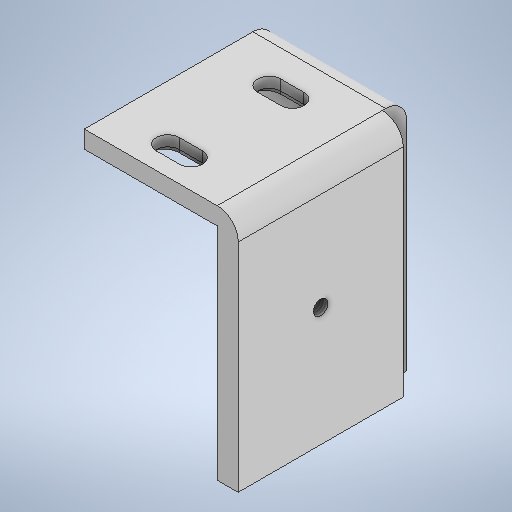
# Autodesk Inventor part: TS_Adapter_Greifer_int
Saved by Autodesk Inventor 2025.1 (Build 291241000, 241)
## iProperties
Created: 2025-06-16
Part Number: TS_Adapter_Greifer_int
Material: Generisch
Document SubType Name: Modeling
Designer: tino
Density: 1 g/cm^3
Appearance: Vorgabe
Author: tino
Autodesk Inventor part; units mm, degrees
ref_plane "YZ Plane" through (0, 0, 0) normal (1, 0, 0) x (0, 1, 0)
ref_plane "XZ Plane" through (0, 0, 0) normal (0, 1, 0) x (-1, 0, 0)
ref_plane "XY Plane" through (0, 0, 0) normal (0, 0, 1) x (1, 0, 0)
sketch "Skizze1" plane through (0, 0, 0) normal (0, 0, 1) x (1, 0, 0)
  line L0 (-19, 27.1) -> (19, 27.1)
  line L1 (19, 27.1) -> (19, -27.1)
  line L2 (19, -27.1) -> (-19, -27.1)
  line L3 (-19, -27.1) -> (-19, 27.1)
  line L4 (0, 37.94) -> (0, -37.94) projected
  line L5 (-26.6, 0) -> (26.6, 0) projected
  point P0 (0, 0)
  dimension "d0" = 38
  dimension "d1" = 54.2
  dimension "d46" = 19
  dimension "d47" = 27.1
  constraints: 8 end point, 2 parallel, 1 horizontal, 1 perpendicular
  measures "d0" distance of L1.end L2.end
  measures "d1" distance of L2.end L0.start
  measures "d46" distance between parallel lines of L3 L4
  measures "d47" distance between parallel lines of L5 L2
extrude "Extrusion1" add sketch "Skizze1" along normal blind 63
sketch "Skizze2" plane through (0, 0, 63) normal (0, 0, 1) x (1, 0, 0)
  line L0 (-19, -27.1) -> (19, -27.1) projected
  line L1 (-19, -27.1) -> (19, -27.1)
  line L2 (19, -27.1) -> (19, 21.1)
  line L3 (19, 21.1) -> (-19, 21.1)
  line L4 (-19, 21.1) -> (-19, -27.1)
  line L5 (-19, 27.1) -> (-19, -27.1) projected
  line L6 (19, 27.1) -> (-19, 27.1) projected
  point P0 (0, 0)
  dimension "d4" = 38
  dimension "d6" = 6
  constraints: 8 end point, 2 parallel, 1 collinear, 1 horizontal, 1 perpendicular, 1 point on line
  measures "d4" distance of L2.end L3.end
  measures "d6" distance between parallel lines of L6 L3
extrude "Extrusion2" cut sketch "Skizze2" against normal through all
sketch "Skizze6" plane through (-19, 27.1, 0) normal (0, 1, 0) x (1, 0, 0)
  line L0 (38, -63) -> (0, -63) projected
  line L1 (38, 0) -> (0, 0) projected
  line L2 (19, 12.6) -> (19, -75.6) projected
  point P0 (19, 0)
  point P1 (19, -44)
  point P2 (19, -19)
  dimension "d48" = 25
  dimension "d49" = 63
  dimension "d50" = 19
  constraints: 1 point on line, 1 vertical alignment
  measures "d48" distance of point (19, -19) point (19, -44)
  measures "d49" distance between parallel lines of L0 L1
  measures "d50" distance from line of L1 point (19, -19)
hole "Bohrung4" at (0, 27.1, 44) at (0, 27.1, 19) direction (0, -1, 0) diameter 5 depth 2.5
sketch "Skizze13" plane through (-19, 21.1, 63) normal (0, -1, 0) x (1, 0, 0)
  line L0 (38, 0) -> (38, -63) projected
  line L1 (0, -63) -> (0, 0) projected
  line L2 (38, -63) -> (0, -63) projected
  line L3 (0, 0) -> (38, 0) projected
  point P0 (19, -63)
  point P1 (7.6, -21.5)
  point P2 (27.6, -21.5)
  point P3 (27.6, -41.5)
  point P4 (7.6, -41.5)
  dimension "d102" = 20
  dimension "d103" = 20
  dimension "d104" = 38
  dimension "d105" = 7.6
  dimension "d106" = 63
  dimension "d107" = 21.5
  constraints: 2 horizontal alignment, 2 vertical alignment
  measures "d102" distance of point (27.6, -21.5) point (7.6, -21.5)
  measures "d103" distance of point (27.6, -21.5) point (27.6, -41.5)
  measures "d104" distance between parallel lines of L0 L1
  measures "d105" distance from line of L1 point (7.6, -41.5)
  measures "d106" distance between parallel lines of L2 L3
  measures "d107" distance from line of L2 point (27.6, -41.5)
hole "Bohrung6" at (-11.4, 21.1, 41.5) at (8.6, 21.1, 41.5) at (8.6, 21.1, 21.5) at (-11.4, 21.1, 21.5) direction (0, 1, 0) diameter 4.5 end through all counterbore diameter 8 counterbore depth 4 clearance for "Innensechskantkopfschraube" size "M4" standard "ANSI Metrisches M Profil"
sketch "Skizze14" plane through (0, 0, 63) normal (0, 0, 1) x (1, 0, 0)
  line L0 (19, 27.1) -> (-19, 27.1) projected
  line L1 (-19, 27.1) -> (19, 27.1)
  line L2 (19, 27.1) -> (19, -27.1)
  line L3 (19, -27.1) -> (-19, -27.1)
  line L4 (-19, -27.1) -> (-19, 27.1)
  line L5 (19, 21.1) -> (19, 27.1) projected
  point P0 (0, 0)
  dimension "d115" = 54.2
  constraints: 8 end point, 2 parallel, 1 collinear, 1 horizontal, 1 perpendicular
  measures "d115" distance between parallel lines of L0 L3
extrude "Extrusion8" add sketch "Skizze14" along normal blind 5
sketch "Skizze15" plane through (0, 0, 68) normal (0, 0, -1) x (-1, 0, 0)
  line L0 (-19, 21.1) -> (19, 21.1) projected
  line L1 (3.3, 13.4) -> (-3.3, 13.4)
  line L2 (-3.3, 13.4) -> (-3.3, 6.8)
  line L3 (-3.3, 6.8) -> (3.3, 6.8)
  line L4 (3.3, 6.8) -> (3.3, 13.4)
  line L5 (3.3, 13.4) -> (-3.3, 6.8) construction
  line L6 (-3.3, 13.4) -> (3.3, 6.8) construction
  arc A0 (3.3, 6.8) -> (3.3, 13.4) centre (3.3, 10.1) ccw
  arc A1 (-3.3, 13.4) -> (-3.3, 6.8) centre (-3.3, 10.1) ccw
  line L7 (3.3, -22.2) -> (-3.3, -22.2)
  line L8 (-3.3, -22.2) -> (-3.3, -15.6)
  line L9 (-3.3, -15.6) -> (3.3, -15.6)
  line L10 (3.3, -15.6) -> (3.3, -22.2)
  line L11 (3.3, -22.2) -> (-3.3, -15.6) construction
  line L12 (-3.3, -22.2) -> (3.3, -15.6) construction
  arc A2 (3.3, -22.2) -> (3.3, -15.6) centre (3.3, -18.9) ccw
  arc A3 (-3.3, -15.6) -> (-3.3, -22.2) centre (-3.3, -18.9) ccw
  point P0 (0, 0)
  point P1 (0, 10.1)
  point P2 (0, -18.9)
  dimension "d118" = 11
  dimension "d119" = 29
  dimension "d149" = 6.6
  dimension "d150" = 6.6
  dimension "d151" = 6.6
  dimension "d152" = 6.6
  dimension "d153" = 3.3
  constraints: 24 end point, 8 point on circle, 6 tangent, 4 centre point, 4 midpoint, 4 parallel, 2 horizontal, 2 perpendicular, 2 vertical alignment
  measures "d118" distance from line of point (0, 10.1) L0
  measures "d119" distance of point (0, -18.9) point (0, 10.1)
  measures "d149" distance of L3.end L2.end
  measures "d150" distance of L2.end L1.end
  measures "d151" distance of L8.end L9.end
  measures "d152" distance of L7.end L8.end
  measures "d153" radius of A2
sketch "Sketch17" plane through (19, 21.1, 0) normal (1, 0, 0) x (0, 0, -1)
  line L0 (-68, -48.2) -> (0, -48.2)
  line L1 (0, -48.2) -> (0, -1)
  line L2 (0, -1) -> (-68, -1)
  line L3 (-68, -1) -> (-68, -48.2)
  line L4 (-63, 0) -> (0, 0) projected
  dimension "d137" = 1
  constraints: 8 end point, 2 parallel, 1 horizontal, 1 perpendicular
  measures "d137" distance between parallel lines of L4 L2
extrude "Extrusion9" add sketch "Sketch17" along normal blind 6
fillet "Fillet2" radius 6 2 edges at (25, -3.5, 68) (0, 27.1, 68)
sketch "Sketch18" plane through (25, 21.1, 0) normal (1, 0, 0) x (0, 0, -1)
  line L0 (-62, -48.2) -> (0, -48.2) projected
  line L1 (0, -1) -> (-62, -1) projected
  point P0 (0, -21.1)
  point P1 (-34.0313, -24.6)
  dimension "d139" = 23.6
  dimension "d140" = 47.2
  measures "d139" distance from line of L0 point (-34.031, -24.6)
  measures "d140" distance between parallel lines of L1 L0
hole "Hole9" at (25, -3.5, 34.0313) direction (-1, 0, 0) diameter 4.134 end through all thread size "M5x0.8" class "6H" standard "ISO Metric profile"
extrude "Extrusion10" cut sketch "Skizze15" along normal blind 6
sketch "Sketch19" plane through (0, 0, 63) normal (0, 0, -1) x (-1, 0, 0)
  arc A0 (3.3, -22.2) -> (3.3, -15.6) centre (3.3, -18.9) ccw projected
  line L0 (3.3, -22.2) -> (-3.3, -22.2) projected
  arc A1 (-3.3, -15.6) -> (-3.3, -22.2) centre (-3.3, -18.9) ccw projected
  line L1 (-3.3, -15.6) -> (3.3, -15.6) projected
  line L2 (-3.3, 13.4) -> (3.3, 13.4) projected
  arc A2 (3.3, 6.8) -> (3.3, 13.4) centre (3.3, 10.1) ccw projected
  line L3 (3.3, 6.8) -> (-3.3, 6.8) projected
  arc A3 (-3.3, 13.4) -> (-3.3, 6.8) centre (-3.3, 10.1) ccw projected
  line L4 (19, 21.1) -> (-19, 21.1) projected
  line L5 (-19, 20.1) -> (-19, 21.1) projected
  line L6 (-19, -27.1) -> (-19, 20.1) projected
  line L7 (19, -27.1) -> (-19, -27.1) projected
  line L8 (19, 21.1) -> (19, -27.1) projected
  line L9 (-9.0001, 14.625) -> (8.9999, 14.625)
  line L10 (8.9999, 14.625) -> (8.9999, 5.625)
  line L11 (8.9999, 5.625) -> (-9.0001, 5.625)
  line L12 (-9.0001, 5.625) -> (-9.0001, 14.625)
  line L13 (-9.0001, 14.625) -> (8.9999, 5.625) construction
  line L14 (8.9999, 14.625) -> (-9.0001, 5.625) construction
  circle A4 centre (4.4999, 10.125) radius 4.5
  circle A5 centre (-4.5001, 10.125) radius 4.5
  line L15 (-9.0001, -14.4) -> (8.9999, -14.4)
  line L16 (8.9999, -14.4) -> (8.9999, -23.4)
  line L17 (8.9999, -23.4) -> (-9.0001, -23.4)
  line L18 (-9.0001, -23.4) -> (-9.0001, -14.4)
  line L19 (-9.0001, -14.4) -> (8.9999, -23.4) construction
  line L20 (8.9999, -14.4) -> (-9.0001, -23.4) construction
  circle A6 centre (4.4999, -18.9) radius 4.5
  circle A7 centre (-4.5001, -18.9) radius 4.5
  arc A8 (-3.3, -15.6) -> (-3.3, -22.2) centre (-3.3, -18.9) ccw projected
  point P0 (0, 0)
  point P1 (-0.0001, 10.125)
  point P2 (-0.1415, -24.1318)
  point P3 (-0.0001, -18.9)
  point P4 (-0.1415, -22.2)
  point P5 (-4.5001, -23.4)
  point P6 (4.4999, -23.4)
  point P7 (4.4999, -14.4)
  point P8 (-4.5001, -14.4)
  point P9 (-4.5001, 5.625)
  point P10 (4.4999, 5.625)
  point P11 (4.4999, 14.625)
  point P12 (-4.5001, 14.625)
  dimension "d156" = 18
  dimension "d157" = 9
  dimension "d158" = 9
  dimension "d160" = 18
  dimension "d161" = 9
  dimension "d162" = 9
  dimension "d165" = 9
  dimension "d166" = 1.2001
  dimension "d167" = 1.2001
  constraints: 24 end point, 7 tangent, 4 centre point, 4 midpoint, 4 parallel, 2 horizontal, 2 perpendicular, 1 point on line
  measures "d156" distance of L10.end L11.end
  measures "d157" distance of L9.end L10.end
  measures "d158" diameter of A4
  measures "d160" distance of L17.start L17.end
  measures "d161" distance of L16.start L17.start
  measures "d162" diameter of A6
  measures "d165" diameter of A7
  measures "d166" horizontal distance of A3.centre A5.centre
  measures "d167" distance of A1.centre A7.centre
extrude "Extrusion11" cut sketch "Sketch19" against normal blind 2 contours A0 L1 A6 L0 | A6 L17 A7 L0 | L1 A7 L15 A6 | A7 L1 A1 L0 | A3 L3 A5 L2 | A5 L9 A4 L2 | A4 L3 A2 L2 | L3 A4 L11 A5 picked at (8.1543, -18.4336) picked at (-8.1544, -18.4336) picked at (-8.1544, 10.583) picked at (8.1543, 10.583)
equation "\"d46\" = 0.5 * d0"
equation "\"d47\" = 0.5 * d1"
equation "\"d50\" = -0.5 * d48 + 0.5 * d49"
equation "\"d107\" = -0.5 * d103 + 0.5 * d106"
equation "\"d139\" = 0.5 * d140"
equation "\"d167\" = d166"
